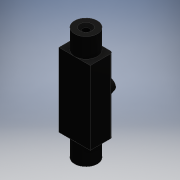
# Autodesk Inventor part: tracks_center_sod_ii
Saved by Autodesk Inventor 2016 (Build 200138000, 138)
## iProperties
Created: 2016-11-04
Part Number: tracks_center_sod_ii
Material: Generic
Document SubType Name: Modeling
Designer: hesaon
Density: 1 g/cm^3
Appearance: Default
Author: hesaon
Autodesk Inventor part; units mm, degrees
ref_plane "YZ Plane" through (0, 0, 0) normal (1, 0, 0) x (0, 1, 0)
ref_plane "XZ Plane" through (0, 0, 0) normal (0, 1, 0) x (-1, 0, 0)
ref_plane "XY Plane" through (0, 0, 0) normal (0, 0, 1) x (1, 0, 0)
sketch "Sketch1" plane through (0, 0, 0) normal (0, 1, 0) x (-1, 0, 0)
  line L0 (0, 0) -> (11.7, 0)
  line L1 (11.7, 0) -> (11.7, -42)
  line L2 (11.7, -42) -> (0, -42)
  line L3 (0, -42) -> (0, 0)
  dimension "p" = 11.7
  dimension "d1" = 42
  constraints: 8 end point, 2 parallel, 1 horizontal, 1 perpendicular
  measures "p" distance of L1.end L2.end
  measures "d1" distance of L1.end L0.end
extrude "Extrusion1" add sketch "Sketch1" along normal blind 8.5
sketch "Sketch2" plane through (-11.7, 0, 0) normal (0, 0, 1) x (1, 0, 0)
  circle A0 centre (5.85, 4.25) radius 1.25
  line L0 (0, 8.5) -> (11.7, 8.5) projected
  line L1 (0, 0) -> (0, 8.5) projected
  point P0 (11.7, 0)
  dimension "d4" = 2.5
  dimension "d5" = 4.25
  dimension "d6" = 5.85
  constraints: 1 centre point
  measures "d4" diameter of A0
  measures "d5" distance from line of L0 A0.centre
  measures "d6" distance from line of L1 A0.centre
extrude "Extrusion2" cut sketch "Sketch2" against normal through all
sketch "Sketch3" plane through (-11.7, 0, 0) normal (0, 0, 1) x (1, 0, 0)
  circle A0 centre (5.85, 4.25) radius 1.25 projected
  circle A1 centre (5.85, 4.25) radius 4.25
  line L0 (11.7, 8.5) -> (0, 8.5) projected
  line L1 (0, 8.5) -> (11.7, 8.5)
  line L2 (11.7, 0) -> (11.7, 8.5) projected
  line L3 (11.7, 8.5) -> (11.7, 0)
  line L4 (0, 0) -> (11.7, 0) projected
  line L5 (11.7, 0) -> (0, 0)
  line L6 (0, 0) -> (0, 8.5) projected
  line L7 (0, 0) -> (0, 8.5)
  dimension "RD" = 8.5
  constraints: 8 end point, 3 collinear, 1 centre point, 1 coincident, 1 horizontal
  measures "RD" diameter of A1
extrude "Extrusion3" cut sketch "Sketch3" against normal blind 7.3 contours A1 L0 L2 L4 | A1 L4 L6 L0
sketch "Sketch4" plane through (0, 0, -42) normal (0, 0, -1) x (-1, 0, 0)
  circle A0 centre (5.85, 4.25) radius 1.25 projected
  circle A1 centre (5.85, 4.25) radius 4.25
  line L0 (0, 8.5) -> (11.7, 8.5) projected
  line L1 (11.7, 0) -> (0, 0) projected
  line L2 (0, 8.5) -> (0, 0)
  line L3 (0, 0) -> (11.7, 0)
  line L4 (11.7, 0) -> (11.7, 8.5)
  line L5 (11.7, 8.5) -> (0, 8.5)
  dimension "d12" = 8.5
  constraints: 8 end point, 2 perpendicular, 1 centre point, 1 coincident, 1 collinear, 1 vertical
  measures "d12" diameter of A1
extrude "Extrusion4" cut sketch "Sketch4" against normal blind 7.3 contours A1 L0 L4 L1 | A1 L1 L2 L0
sketch "Sketch5" plane through (0, 8.5, 0) normal (0, 1, 0) x (1, 0, 0)
  line L0 (-11.7, 7.3) -> (-11.7, 34.7) projected
  line L1 (0, 34.7) -> (0, 7.3) projected
  line L2 (-1, 23) -> (-10.7, 23)
  line L3 (-10.7, 19) -> (-1, 19)
  line L4 (-10.7, 19) -> (-10.7, 23)
  line L5 (-1, 19) -> (-1, 23)
  point P0 (0, 0)
  dimension "d19" = 4
  dimension "d20" = 4
  dimension "d21" = 9.7
  dimension "d22" = 1
  dimension "d23" = 19
  constraints: 8 end point, 2 perpendicular
  measures "d19" distance of L2.start L3.end
  measures "d20" distance of L2.end L3.start
  measures "d21" distance of L3.end L3.start
  measures "d22" distance between parallel lines of L0 L4
  measures "d23" distance from line of point (0, 0) L3
extrude "Extrusion5" add sketch "Sketch5" along normal blind 3
sketch "Sketch6" plane through (-1, 8.5, -23) normal (0, 0, -1) x (-1, 0, 0)
  line L0 (9.7, 3) -> (0, 3) projected
  line L1 (9.7, 3) -> (8.7, 3)
  line L2 (0, 0) -> (9.7, 0) projected
  line L3 (8.7, 3) -> (9.7, 0)
  line L4 (9.7, 0) -> (9.7, 3)
  line L5 (0, 3) -> (1, 3)
  line L6 (1, 3) -> (0, 0)
  line L7 (0, 0) -> (0, 3)
  point P0 (-1, -8.5)
  dimension "d26" = 1
  dimension "d27" = 1
  constraints: 12 end point, 2 perpendicular, 2 point on line
  measures "d26" distance of L0.start L1.end
  measures "d27" distance of L0.end L5.end
extrude "Extrusion6" cut sketch "Sketch6" against normal through all contours L4 L3 L0 | L6 L7 L0
fillet "Fillet1" radius 2 4 edges at (-1.5, 10, -19) (-1.5, 10, -23) (-10.2, 10, -19) (-10.2, 10, -23)
fillet "Fillet2" radius 1 2 edges at (0, 8.5, -21) (-11.7, 8.5, -21)
chamfer "Chamfer1" distance 1 angle 45 2 edges at (-7.1, 4.25, -42) (-7.1, 4.25, 0)
equation "\"d6\" = 0.5 * p"
equation "\"d12\" = RD"
body "Solid1"
